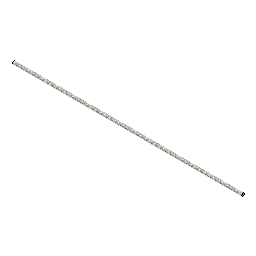
Stainless Steel Rod (Autodesk Fusion 360 design; units mm, degrees)
Autodesk Fusion 360 part; units mm, degrees
sketch "Eskiz1" plane through (0, 0, 0) normal (1, 0, 0) x (0, 0, -1)
  circle A0 centre (0, 0) radius 4
  dimension "d1" = 8
  constraint coincident A0.centre origin
  measures "d1" diameter of A0
extrude "Ekstrüde Et1" add sketch "Eskiz1" along normal blind 700
thread "Diş1" "ISO Metric profile 8.0 M8x0.8 6g" major diameter 7.901 minor diameter 6.9838 pitch 0.8 angle 60 resizes the face on face at (233.3333, -0.9225, -3.8922)
chamfer "Oluk2" distance 3.9 angle 45 1 faces at (0, 0.7523, -0.0139)
